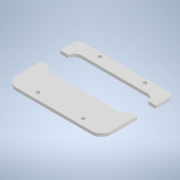
# Autodesk Inventor part: spacer top
Saved by Autodesk Inventor 2022 (Build 260153000, 153)
## iProperties
Created: 2021-06-21
Part Number: spacer top
Material: Generic
Document SubType Name: Modeling
Designer: benka
Density: 1 g/cm^3
Appearance: Default
Author: benka
Autodesk Inventor part; units mm, degrees
ref_plane "YZ Plane" through (0, 0, 0) normal (1, 0, 0) x (0, 1, 0)
ref_plane "XZ Plane" through (0, 0, 0) normal (0, 1, 0) x (-1, 0, 0)
ref_plane "XY Plane" through (0, 0, 0) normal (0, 0, 1) x (1, 0, 0)
sketch "Sketch2" plane through (-170.3284, 0, 65.1839) normal (0, 1, 0) x (-1, 0, 0)
  line L0 (-194.2202, -67.6262) -> (-191.2126, -67.6262)
  line L1 (-276.2126, -67.6262) -> (-273.6697, -67.6262)
  arc A0 (-266.7109, -62.5378) -> (-273.6697, -67.6262) centre (-266.7109, -69.8403) ccw
  line L2 (-201.1789, -62.5378) -> (-266.7109, -62.5378)
  arc A1 (-194.2202, -67.6262) -> (-201.1789, -62.5378) centre (-201.1789, -69.8403) ccw
  arc A2 (-273.9303, -86.3444) -> (-266.7109, -92.5479) centre (-266.7109, -85.2454) ccw
  line L3 (-201.1789, -92.5479) -> (-266.7109, -92.5479)
  line L4 (-191.2128, -86.3444) -> (-193.9596, -86.3444)
  line L5 (-186.2128, -99.4479) -> (-186.2128, -96.4479)
  arc A3 (-191.2128, -104.4479) -> (-186.2128, -99.4479) centre (-191.2128, -99.4479) ccw
  line L6 (-276.2128, -104.4479) -> (-191.2128, -104.4479)
  arc A4 (-281.2128, -99.4479) -> (-276.2128, -104.4479) centre (-276.2128, -99.4479) ccw
  line L7 (-273.9303, -86.3444) -> (-276.2128, -86.3444)
  line L8 (-281.2128, -96.4479) -> (-281.2128, -99.4479)
  line L9 (-186.2128, -96.4479) -> (-186.2128, -86.3444)
  line L10 (-186.2128, -86.3444) -> (-191.2128, -86.3444)
  line L11 (-276.2128, -86.3444) -> (-281.2128, -86.3444)
  line L12 (-281.2128, -86.3444) -> (-281.2128, -96.4479)
  line L13 (-276.2126, -67.6262) -> (-281.2128, -67.6262)
  line L14 (-281.2128, -67.6262) -> (-281.2126, -57.5226)
  line L15 (-191.2126, -67.6262) -> (-186.2128, -67.6262)
  line L16 (-186.2126, -57.5226) -> (-186.2128, -67.6262)
  arc A5 (-201.1789, -92.5479) -> (-193.9596, -86.3444) centre (-201.1789, -85.2454) ccw
  circle A6 centre (-211.2128, -100.4479) radius 2
  circle A7 centre (-256.2128, -100.4479) radius 2
  circle A8 centre (-256.2128, -38.7981) radius 2
  circle A9 centre (-211.2128, -38.7981) radius 2
  arc A10 (-271.2126, -32.4132) -> (-281.2126, -42.4132) centre (-271.2126, -42.4132) ccw
  line L17 (-281.2126, -42.4132) -> (-281.2126, -57.5226)
  line L18 (-196.2126, -32.4132) -> (-271.2126, -32.4132)
  arc A11 (-186.2126, -42.4132) -> (-196.2126, -32.4132) centre (-196.2126, -42.4132) ccw
  line L19 (-186.2126, -57.5226) -> (-186.2126, -42.4132)
  constraints: 40 end point, 16 point on circle, 12 centre point, 8 horizontal, 5 vertical, 4 point on line, 3 perpendicular, 48 other
extrude "Extrusion1" add sketch "Sketch2" along normal blind 3
body "Solid1"
